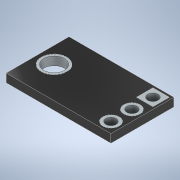
# Autodesk Inventor part: QTR1A_Board
Saved by Autodesk Inventor 2021 (Build 250183000, 183)
## iProperties
Created: 2021-05-13
Part Number: QTR1A_Board
Material: Generic
Document SubType Name: Modeling
Designer: ermoz
Density: 1 g/cm^3
Appearance: Default
Author: ermoz
Autodesk Inventor part; units mm, degrees
ref_plane "YZ Plane" through (0, 0, 0) normal (1, 0, 0) x (0, 1, 0)
ref_plane "XZ Plane" through (0, 0, 0) normal (0, 1, 0) x (-1, 0, 0)
ref_plane "XY Plane" through (0, 0, 0) normal (0, 0, 1) x (1, 0, 0)
sketch "Sketch1" plane through (0, 0, 0) normal (0, 1, 0) x (-1, 0, 0)
  line L0 (-6.35, 3.81) -> (6.35, 3.81)
  line L1 (6.35, 3.81) -> (6.35, -3.81)
  line L2 (6.35, -3.81) -> (-6.35, -3.81)
  line L3 (-6.35, -3.81) -> (-6.35, 3.81)
  line L4 (-6.35, 3.81) -> (6.35, -3.81) construction
  line L5 (6.35, 3.81) -> (-6.35, -3.81) construction
  point P0 (0, 0)
  dimension "d0" = 12.7
  dimension "d1" = 7.62
  constraints: 12 end point, 2 midpoint, 2 parallel, 1 horizontal, 1 perpendicular
  measures "d0" distance of L1.end L2.end
  measures "d1" distance of L0.end L1.end
extrude "Extrusion1" add sketch "Sketch1" along normal blind 1.02
sketch "Sketch2" plane through (0, 1.02, 0) normal (0, 1, 0) x (1, 0, 0)
  circle A0 centre (-4.35, 0) radius 1.25
  circle A1 centre (-4.35, 0) radius 1.55
  circle A2 centre (5.08, 2.54) radius 0.625
  line L0 (4.08, 3.54) -> (6.08, 3.54)
  line L1 (6.08, 3.54) -> (6.08, 1.54)
  line L2 (6.08, 1.54) -> (4.08, 1.54)
  line L3 (4.08, 1.54) -> (4.08, 3.54)
  line L4 (4.08, 3.54) -> (6.08, 1.54) construction
  line L5 (6.08, 3.54) -> (4.08, 1.54) construction
  circle A3 centre (5.08, 0) radius 0.625
  circle A4 centre (5.08, 0) radius 1
  circle A5 centre (5.08, -2.54) radius 0.625
  circle A6 centre (5.08, -2.54) radius 1
  line L6 (0, 0) -> (2.2698, 0)
  line L7 (6.35, -3.81) -> (6.35, 3.81) projected
  line L8 (-6.35, 3.81) -> (-6.35, -3.81) projected
  dimension "d4" = 2.5
  dimension "d5" = 0.3
  dimension "d7" = 2
  dimension "d8" = 2.54
  dimension "d9" = 1.27
  dimension "d10" = 1.25
  dimension "d15" = 2
  constraints: 14 end point, 7 centre point, 3 equal radius, 3 midpoint, 2 coincident, 2 horizontal, 2 parallel, 2 perpendicular, 2 tangent, 2 vertical alignment, 1 horizontal alignment, 1 symmetric about line
  measures "d4" diameter of A0
  measures "d5" radial gap between concentric circles of A0 A1
  measures "d7" diameter of A4
  measures "d8" distance of A3.centre A2.centre
  measures "d9" distance from line of L7 A2.centre
  measures "d10" diameter of A3
  measures "d15" distance from line of L8 A0.centre
extrude "Extrusion2" cut sketch "Sketch2" against normal through all contours A0 | A1 | A2 | L0 L1 L2 L3 | A3 | A4 | A5 | A6
extrude "Extrusion3" add sketch "Sketch2" against normal up to surface (1.02 mm away) separate body
body "Solid1"
body "Solid2"
